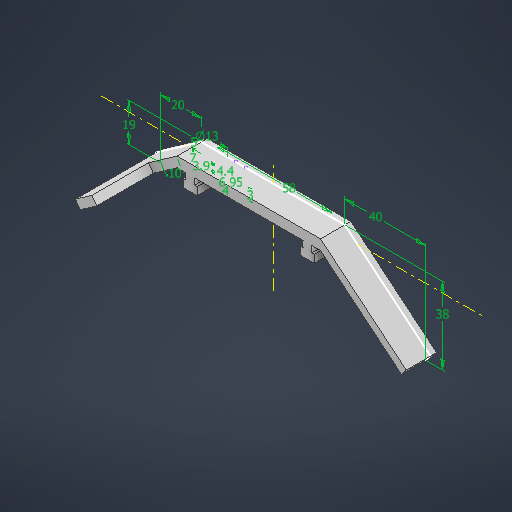
# Autodesk Inventor part: UnitreeGO2_railmount
Saved by Autodesk Inventor 2026.1 (Build 301233000, 233)
## iProperties
Created: 2026-01-16
Part Number: UnitreeGO2_railmount
Material: Generic
Document SubType Name: Modeling
Designer: aimot
Density: 1 g/cm^3
Appearance: Default
Author: aimot
Autodesk Inventor part; units mm, degrees
ref_plane "YZ Plane" through (0, 0, 0) normal (1, 0, 0) x (0, 1, 0)
ref_plane "XZ Plane" through (0, 0, 0) normal (0, 1, 0) x (-1, 0, 0)
ref_plane "XY Plane" through (0, 0, 0) normal (0, 0, 1) x (1, 0, 0)
sketch "Sketch2" plane through (0, 0, 0) normal (0, 0, 1) x (1, 0, 0)
  line L0 (-32.475, -3.1) -> (-25.525, -3.1)
  line L1 (-25.525, -3.1) -> (-25.525, -7)
  line L2 (-25.525, -7) -> (-32.475, -7)
  line L3 (-32.475, -7) -> (-32.475, -3.1)
  line L4 (-31.2, 0) -> (-26.8, 0)
  line L5 (-26.8, 0) -> (-26.8, -3.1)
  line L6 (-26.8, -3.1) -> (-31.2, -3.1)
  line L7 (-31.2, -3.1) -> (-31.2, 0)
  line L8 (-35.5, 0) -> (0, 0)
  line L9 (0, 5) -> (-35.5, 5)
  line L10 (-35.5, 5) -> (-35.5, 0)
  line L11 (-29, 6.5254) -> (-29, -10.3092) construction
  line L12 (0, -40.9051) -> (0, 14.4305) construction
  line L13 (32.475, -3.1) -> (25.525, -3.1)
  line L14 (25.525, -3.1) -> (25.525, -7)
  line L15 (25.525, -7) -> (32.475, -7)
  line L16 (32.475, -7) -> (32.475, -3.1)
  line L17 (31.2, 0) -> (26.8, 0)
  line L18 (26.8, 0) -> (26.8, -3.1)
  line L19 (26.8, -3.1) -> (31.2, -3.1)
  line L20 (31.2, -3.1) -> (31.2, 0)
  line L21 (35.5, 0) -> (0, 0)
  line L22 (0, 5) -> (35.5, 5)
  line L23 (35.5, 5) -> (35.5, 0)
  line L24 (29, 6.5254) -> (29, -10.3092) construction
  line L25 (-85.0097, 0) -> (105.1151, 0) construction
  line L26 (35.5, 5) -> (77.9544, -30.0249)
  line L27 (77.9544, -30.0249) -> (75.5, -33)
  line L28 (75.5, -33) -> (35.5, 0)
  line L29 (-35.5, 5) -> (35.5, 5)
  line L30 (35.5, 5) -> (35.5, -7)
  line L31 (35.5, -7) -> (-35.5, -7)
  line L32 (-35.5, -7) -> (-35.5, 5)
  line L33 (-35.5, 5) -> (-57.849, -10.6443)
  line L34 (-57.849, -10.6443) -> (-55.5, -14)
  line L35 (-55.5, -14) -> (-35.5, 0)
  line L36 (-49.6567, -4.9097) -> (-47.3077, -8.2654)
  line L37 (-21.525, -7) -> (-21.525, -4)
  line L38 (-21.525, -4) -> (0, -4)
  line L39 (21.525, -7) -> (21.525, -4)
  line L40 (21.525, -4) -> (0, -4)
  line L41 (-35.5, -7) -> (-45.5, -7)
  line L42 (35.5, -7) -> (43.9848, -7)
  point P0 (-13.25, 5)
  point P1 (-18.25, 5)
  point P2 (29, -7)
  dimension "d1" = 4.4
  dimension "d2" = 6.95
  dimension "d3" = 3.9
  dimension "d4" = 5
  dimension "d5" = 58
  dimension "d6" = 7
  dimension "d7" = 13
  dimension "d28" = 38
  dimension "d29" = 40
  dimension "d30" = 20
  dimension "d31" = 19
  dimension "d32" = 10
  dimension "d37" = 4
  dimension "d38" = 3
  constraints: 82 end point, 14 point on line, 14 symmetric about line, 9 parallel, 8 perpendicular, 5 horizontal, 2 midpoint, 1 collinear, 1 vertical, 2 other
  measures "d1" distance between parallel lines of L5 L7
  measures "d2" distance between parallel lines of L1 L3
  measures "d3" distance between parallel lines of L2 L0
  measures "d4" distance between parallel lines of L9 L8
  measures "d5" distance between parallel lines of L24 L11
  measures "d6" distance between parallel lines of L8 L2
  measures "d7" diameter of L10 L11
  measures "d28" vertical distance of L23.start L27.end
  measures "d29" horizontal distance of L27.end L23.start
  measures "d30" horizontal distance of L34.end L9.end
  measures "d31" vertical distance of L9.end L34.end
  measures "d32" distance between parallel lines of L36 L34
  measures "d37" distance between parallel lines of L37 L1
  measures "d38" distance between parallel lines of L38 L31
extrude "Extrusion1" add sketch "Sketch2" along normal blind 12 contours L0 L1 L2 L3 | L7 L4 L5 L0 | L8 L10 L9 L22 L23 L21 L17 L4 | L35 L36 L33 L10 | L17 L20 L13 L18 | L14 L13 L16 L15 | L26 L27 L28 L23
extrude "Extrusion2" add sketch "Sketch2" along normal blind 40 contours L35 L34 L33 L36
extrude "Extrusion3" add sketch "Sketch2" against normal blind 3 contours L3 L31 L32 L8 L7 L0 | L0 L1 L2 L3 | L7 L4 L5 L0 | L5 L8 L21 L18 L13 L14 L31 L39 L40 L38 L37 L1 L0 | L8 L10 L9 L22 L23 L21 L17 L4 | L41 L35 L32 | L35 L36 L33 L10 | L35 L34 L33 L36 | L17 L20 L13 L18 | L14 L13 L16 L15 | L21 L30 L31 L16 L13 L20 | L26 L27 L28 L23 | L28 L42 L30
body "Solid1"
